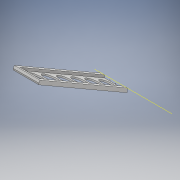
# Autodesk Inventor part: V2
Saved by Autodesk Inventor 2018 (Build 220112000, 112)
## iProperties
Created: 2019-04-27
Part Number: V2
Material: Genérico
Document SubType Name: Modeling
Designer: EDWIN
Density: 1 g/cm^3
Appearance: Valor por defecto
Author: EDWIN
Autodesk Inventor part; units mm, degrees
sketch "Boceto1" plane through (0, 0, 0) normal (0, 0, 1) x (1, 0, 0)
  line L0 (81, 20) -> (81, 63.5)
  line L1 (-27.5, 63.5) -> (-27.5, -5)
  line L2 (-27.5, -5) -> (16, -5)
  line L3 (16, -5) -> (16, 20)
  line L4 (11, 25) -> (11, -5)
  line L5 (-22.5, 58.5) -> (-22.5, -5)
  line L6 (11, 25) -> (81, 25)
  line L7 (-27.5, 63.5) -> (81, 63.5)
  line L8 (-22.5, 58.5) -> (81, 58.5)
  line L9 (16, 20) -> (81, 20)
  point P0 (0, 0)
  dimension "d7" = 5
  dimension "d68" = 5
  dimension "d69" = 33.5
  dimension "d74" = 5
  dimension "d75" = 33.5
  dimension "d76" = 5
  dimension "d77" = 70
  dimension "d111" = 30
  constraints: 20 end point, 4 horizontal, 4 point on line, 3 perpendicular, 1 parallel
  measures "d7" distance between parallel lines of L1 L5
  measures "d68" distance between parallel lines of L4 L3
  measures "d69" distance between parallel lines of L5 L4
  measures "d74" distance between parallel lines of L7 L8
  measures "d75" distance between parallel lines of L6 L8
  measures "d76" distance between parallel lines of L6 L9
  measures "d77" distance between parallel lines of L0 L4
  measures "d111" distance between parallel lines of L6 L2
extrude "Extrusión1" add sketch "Boceto1" against normal blind 2.5
extrude "Extrusión2" add sketch "Boceto1" along normal blind 1 contours L9 L3 L2 L4 L6 L0 | L8 L5 L2 L1 L7 L0
ref_plane "Plano de trabajo3" through (29.25, 58.5, 1) normal (0, 0, 1) x (1, 0, 0)
mirror "Simetría3" about plane through (29.25, 58.5, 1) normal (0, 0, 1) of "Extrusión2", "Extrusión1"
sketch "Boceto6" plane through (-27.5, 63.5, 4.5) normal (0, 0, 1) x (1, 0, 0)
  line L0 (108.5, -43.5) -> (43.5, -43.5) projected
  line L1 (0, -68.5) -> (0, 0) projected
  line L2 (0, -43.5) -> (0, -51.5)
  line L3 (43.5, -43.5) -> (43.5, -68.5) projected
  line L4 (0, -43.5) -> (38.5, -43.5)
  line L5 (38.5, -68.5) -> (38.5, -38.5) projected
  line L6 (0, -51.5) -> (38.5, -51.5)
  line L7 (38.5, -43.5) -> (38.5, -51.5)
  point P0 (27.5, -63.5)
  point P1 (43.5, -51.5)
  dimension "d78" = 8
  constraints: 8 end point, 4 point on line, 1 collinear, 1 horizontal, 1 parallel
  measures "d78" distance of L2.start L2.end
extrude "Extrusión11" cut sketch "Boceto6" against normal blind 4.5
sketch "Boceto7" plane through (-27.5, -5, -2.5) normal (-1, 0, 0) x (0, 0, 1)
  line L0 (0, 0) -> (0, 68.5) projected
  line L1 (0, 0) -> (0, -42.4)
  line L2 (0, 0) -> (7, 0) projected
  line L3 (0, 0) -> (7, 0)
  line L4 (7, 0) -> (7, -42.4)
  line L5 (0, -42.4) -> (86.5, -192.2224)
  line L6 (86.5, -192.2224) -> (89, -192.2224)
  line L7 (89, -192.2224) -> (92.375, -190.2738)
  line L8 (2.5, 0) -> (2.5, -42.4)
  line L9 (0, 0) -> (7, 0) projected
  line L10 (0, 0) -> (2.5, 0)
  line L11 (86.5, -192.2224) -> (89, -192.2224)
  line L12 (89, -192.2224) -> (92.375, -190.2738)
  line L13 (2.5, -42.4) -> (89, -192.2224)
  line L14 (0, -42.4) -> (-1.0904, -42.4)
  line L15 (7, -42.4) -> (92.375, -190.2738)
  line L16 (86.5, -187.8923) -> (89.875, -185.9437)
  point P0 (2.5, 5)
  point P1 (4.5, 0)
  point P2 (-0.5452, -42.4)
  dimension "d81" = 42.4
  dimension "d82" = 173
  dimension "d88" = 120
  dimension "d108" = 5
  constraints: 28 end point, 3 horizontal, 3 perpendicular, 2 collinear, 2 horizontal alignment, 2 parallel, 2 point on line, 1 midpoint, 1 vertical
  measures "d81" distance of L0.start L1.end
  measures "d82" distance of L1.end L5.end
  measures "d88" angle of L5 L14
  measures "d108" distance between parallel lines of L7 L16
ref_plane "Plano de trabajo4" through (-5.75, -5, -2.5) normal (1, 0, 0) x (0, 0, -1)
extrude "Extrusión12" add sketch "Boceto7" against normal blind 21.75 contours L2 L8 L13 L6 L5 L1
extrude "Extrusión13" add sketch "Boceto7" against normal blind 5 contours L2 L4 L15 L16 L13 L8
extrude "Extrusión14" add sketch "Boceto7" against normal blind 21.75 contours L13 L16 L15 L7
mirror "Simetría4" about plane through (-5.75, -5, -2.5) normal (1, 0, 0) of "Extrusión12", "Extrusión13", "Extrusión14"
sketch "Boceto8" plane through (-22.5, -47.4, 0) normal (0, 0.5, 0.866) x (1, 0, 0)
  line L0 (0, 0) -> (33.5, 0) projected
  line L1 (16.75, 0) -> (16.75, -5)
  circle A0 centre (16.75, -15.25) radius 10.25
  line L2 (16.75, -25.5) -> (16.75, -30.5)
  circle A1 centre (16.75, -41.5) radius 11
  line L3 (16.75, -52.5) -> (16.75, -57.5)
  circle A2 centre (16.75, -68.69) radius 11.19
  line L4 (16.75, -79.88) -> (16.75, -84.88)
  circle A3 centre (16.75, -96.38) radius 11.5
  line L5 (16.75, -107.88) -> (16.75, -112.88)
  circle A4 centre (16.75, -125.07) radius 12.19
  line L6 (16.75, -137.26) -> (16.75, -142.26)
  circle A5 centre (16.75, -155.01) radius 12.75
  point P0 (22.5, 41.0496)
  dimension "d105" = 25.5
  dimension "d94" = 5
  dimension "d95" = 20.5
  dimension "d96" = 5
  dimension "d97" = 5
  dimension "d98" = 5
  dimension "d99" = 5
  dimension "d100" = 5
  dimension "d101" = 22
  dimension "d102" = 22.38
  dimension "d103" = 23
  dimension "d104" = 24.38
  constraints: 12 end point, 10 point on circle, 6 vertical, 5 centre point, 1 midpoint, 1 vertical alignment, 2 other
  measures "d94" distance of L1.start L1.end
  measures "d95" diameter of A0
  measures "d96" distance of L2.start L2.end
  measures "d97" distance of L3.start L3.end
  measures "d98" distance of L4.start L4.end
  measures "d99" distance of L5.start L5.end
  measures "d100" distance of L6.start L6.end
  measures "d101" diameter of A1
  measures "d102" diameter of A2
  measures "d103" diameter of A3
  measures "d104" diameter of A4
extrude "Extrusión15" cut sketch "Boceto8" against normal blind 21.75
sketch "Boceto9" plane through (-27.5, 63.5, -2.5) normal (-1, 0, 0) x (0, 0, 1)
  line L0 (2.5, -51.5) -> (2.5, -110.9) projected
  line L1 (0, 0) -> (0, -110.9) projected
  line L2 (0, -110.9) -> (2.5, -110.9)
  line L3 (2.5, -110.9) -> (2.5, -70.9)
  line L4 (2.5, -70.9) -> (0, -70.9)
  line L5 (0, -70.9) -> (0, -110.9)
  line L6 (0, -43.5) -> (0, -110.9) projected
  line L7 (0, -102.4) -> (2.5, -102.4)
  point P0 (2.5, -63.5)
  point P1 (7, -110.9)
  dimension "d109" = 2.5
  dimension "d110" = 40
  dimension "d112" = 31.5
  constraints: 10 end point, 2 parallel, 2 perpendicular, 2 point on line, 1 horizontal
  measures "d109" distance of L1.end L2.end
  measures "d110" distance between parallel lines of L2 L4
  measures "d112" distance between parallel lines of L7 L4
extrude "Extrusión16" cut sketch "Boceto9" against normal through all contours L0 L7 L1 L4
ref_plane "Plano de trabajo5" through (-27.5, -47.4, 0) normal (0, -1, 0) x (1, 0, 0)
ref_plane "Plano de trabajo6" through (-27.5, -47.4, 0) normal (0, -1, 0) x (1, 0, 0)
sketch "Boceto11" plane through (-27.5, -47.4, 0) normal (0, -1, 0) x (1, 0, 0)
  line L0 (43.5, 4.5) -> (38.5, 4.5) projected
  line L1 (38.5, 0) -> (38.5, 4.5) projected
  line L2 (5, 0) -> (38.5, 0) projected
  line L3 (5, 4.5) -> (5, 0) projected
  line L4 (0, 4.5) -> (5, 4.5) projected
  line L5 (0, -2.5) -> (0, 4.5) projected
  line L6 (0, -2.5) -> (43.5, -2.5) projected
  line L7 (43.5, 4.5) -> (43.5, -2.5) projected
  line L8 (0, 0) -> (0, -2.5) projected
  line L9 (43.5, -2.5) -> (43.5, 4.5) projected
  circle A0 centre (2.5, 2) radius 1.25
  line L10 (108.5, 2) -> (5, 2) projected
  circle A1 centre (41, 2) radius 1.25
  circle A2 centre (11.5, -1.25) radius 0.75
  circle A3 centre (21.5, -1.25) radius 0.75
  circle A4 centre (31.5, -1.25) radius 0.75
  point P0 (27.5, 0)
  dimension "d117" = 2.5
  dimension "d118" = 2.5
  dimension "d119" = 38.5
  dimension "d120" = 1.5
  dimension "d121" = 1.5
  dimension "d122" = 1.5
  dimension "d123" = 10
  dimension "d124" = 10
  constraints: 5 centre point, 1 horizontal alignment, 1 point on line
  measures "d117" diameter of A0
  measures "d118" diameter of A1
  measures "d119" distance of A1.centre A0.centre
  measures "d120" diameter of A2
  measures "d121" diameter of A3
  measures "d122" diameter of A4
  measures "d123" distance of A3.centre A2.centre
  measures "d124" distance of A3.centre A4.centre
extrude "Extrusión18" add sketch "Boceto11" along normal blind 2.5 contours A1 L10 | L10 A1 | A0
extrude "Extrusión19" cut sketch "Boceto11" against normal blind 2.5 contours A2 | A3 | A4
sketch "Boceto12" plane through (-27.5, -47.4, 0) normal (0, -1, 0) x (1, 0, 0)
  line L0 (0, -2.5) -> (0, 84) projected
  line L1 (0, 4.5) -> (108.5, 4.5) projected
  line L2 (0, -2.5) -> (108.5, -2.5)
  line L3 (108.5, -2.5) -> (108.5, 4.5)
  line L4 (108.5, 4.5) -> (0, 4.5)
  line L5 (0, 4.5) -> (0, -2.5)
  point P0 (27.5, 0)
  constraints: 8 end point, 2 parallel, 1 horizontal, 1 perpendicular
extrude "Extrusión20" cut sketch "Boceto12" against normal through all
extrude "Extrusión21" add sketch "Boceto11" against normal blind 2.4 contours A2 | A3 | A4
extrude "Extrusión22" cut sketch "Boceto11" along normal blind 2.6 contours A1 L10 | L10 A1 | A0
equation "\"d105\" = UnSol"
equation "\"d94\" = razon"
equation "\"d95\" = diezcen"
equation "\"d96\" = razon"
equation "\"d97\" = razon"
equation "\"d98\" = razon"
equation "\"d99\" = razon"
equation "\"d100\" = razon"
equation "\"d101\" = cincuentacen"
equation "\"d102\" = dossol"
equation "\"d103\" = veintecen"
equation "\"d104\" = cincosol"
equation "\"UnSol\" = 25.5"
equation "\"diezcen\" = 20.5"
equation "\"veintecen\" = 23"
equation "\"cincuentacen\" = 22"
equation "\"dossol\" = 22.38"
equation "\"cincosol\" = 24.38"
equation "\"razon\" = 5"
